Autodesk Fusion 360 part; units mm, degrees
(part 2 of 3)
  line L945 (31.8725, -23.9004) -> (31.8863, -23.9048)
  line L946 (31.8863, -23.9048) -> (31.9005, -23.9089)
  line L947 (31.9005, -23.9089) -> (31.9146, -23.9129)
  line L948 (31.9146, -23.9129) -> (31.9289, -23.9165)
  line L949 (31.9289, -23.9165) -> (31.9431, -23.9199)
  line L950 (31.9431, -23.9199) -> (31.9574, -23.9231)
  line L951 (31.9574, -23.9231) -> (31.9717, -23.9261)
  line L952 (31.9717, -23.9261) -> (31.986, -23.9287)
  line L953 (31.986, -23.9287) -> (32.0006, -23.9311)
  line L954 (32.0006, -23.9311) -> (32.0151, -23.9333)
  line L955 (32.0151, -23.9333) -> (32.0297, -23.9352)
  line L956 (32.0297, -23.9352) -> (32.0442, -23.9369)
  line L957 (32.0442, -23.9369) -> (32.0588, -23.9383)
  line L958 (32.0588, -23.9383) -> (32.0733, -23.9394)
  line L959 (32.0733, -23.9394) -> (32.0881, -23.9403)
  line L960 (32.0881, -23.9403) -> (32.1027, -23.941)
  line L961 (32.1027, -23.941) -> (32.1172, -23.9414)
  line L962 (32.1172, -23.9414) -> (32.1321, -23.9415)
  line L963 (32.1321, -23.9415) -> (57.3336, -23.9415)
  line L964 (57.3336, -23.9415) -> (57.3482, -23.9414)
  line L965 (-0.0202, 22.1566) -> (-0.0403, 22.1571)
  line L966 (-0.0403, 22.1571) -> (-0.0604, 22.158)
  line L967 (-0.0604, 22.158) -> (-0.0806, 22.1592)
  line L968 (-0.0806, 22.1592) -> (-0.1007, 22.1608)
  line L969 (-0.1007, 22.1608) -> (-0.1207, 22.1627)
  line L970 (-0.1207, 22.1627) -> (-0.1408, 22.165)
  line L971 (-0.1408, 22.165) -> (-0.1608, 22.1676)
  line L972 (-0.1608, 22.1676) -> (-0.1807, 22.1706)
  line L973 (-0.1807, 22.1706) -> (-0.2006, 22.1739)
  line L974 (-0.2006, 22.1739) -> (-0.2204, 22.1776)
  line L975 (-0.2204, 22.1776) -> (-0.2402, 22.1816)
  line L976 (-0.2402, 22.1816) -> (-0.2598, 22.186)
  line L977 (-0.2598, 22.186) -> (-0.2794, 22.1907)
  line L978 (-0.2794, 22.1907) -> (-0.299, 22.1957)
  line L979 (-0.299, 22.1957) -> (-0.3184, 22.2011)
  line L980 (-0.3184, 22.2011) -> (-0.3377, 22.2068)
  line L981 (-0.3377, 22.2068) -> (-0.3569, 22.2129)
  line L982 (-0.3569, 22.2129) -> (-0.3761, 22.2193)
  line L983 (-0.3761, 22.2193) -> (-0.3951, 22.226)
  line L984 (-0.3951, 22.226) -> (-0.4139, 22.2331)
  line L985 (-0.4139, 22.2331) -> (-0.4327, 22.2405)
  line L986 (-0.4327, 22.2405) -> (-0.4513, 22.2482)
  line L987 (-0.4513, 22.2482) -> (-0.4698, 22.2562)
  line L988 (-0.4698, 22.2562) -> (-0.4882, 22.2646)
  line L989 (-0.4882, 22.2646) -> (-0.5063, 22.2733)
  line L990 (-0.5063, 22.2733) -> (-0.5244, 22.2823)
  line L991 (-0.5244, 22.2823) -> (-0.5423, 22.2916)
  line L992 (-0.5423, 22.2916) -> (-0.56, 22.3012)
  line L993 (-0.56, 22.3012) -> (-0.5775, 22.3111)
  line L994 (-0.5775, 22.3111) -> (-0.5949, 22.3214)
  line L995 (-0.5949, 22.3214) -> (-0.6121, 22.3319)
  line L996 (-0.6121, 22.3319) -> (-0.6291, 22.3427)
  line L997 (-0.6291, 22.3427) -> (-0.6459, 22.3539)
  line L998 (-0.6459, 22.3539) -> (-0.6625, 22.3653)
  line L999 (-0.6625, 22.3653) -> (-0.6789, 22.377)
  line L1000 (-0.6789, 22.377) -> (-0.6951, 22.389)
  line L1001 (-0.6951, 22.389) -> (-0.7111, 22.4012)
  line L1002 (-0.7111, 22.4012) -> (-0.7269, 22.4138)
  line L1003 (-0.7269, 22.4138) -> (-0.7425, 22.4266)
  line L1004 (-0.7425, 22.4266) -> (-0.7578, 22.4397)
  line L1005 (-0.7578, 22.4397) -> (-0.7729, 22.4531)
  line L1006 (-0.7729, 22.4531) -> (-0.7878, 22.4667)
  line L1007 (-0.7878, 22.4667) -> (-0.8024, 22.4806)
  line L1008 (-0.8024, 22.4806) -> (-0.8168, 22.4947)
  line L1009 (-0.8168, 22.4947) -> (-0.8309, 22.5091)
  line L1010 (-0.8309, 22.5091) -> (-0.8448, 22.5237)
  line L1011 (-0.8448, 22.5237) -> (-0.8584, 22.5386)
  line L1012 (-0.8584, 22.5386) -> (-0.8717, 22.5536)
  line L1013 (-0.8717, 22.5536) -> (-0.8848, 22.569)
  line L1014 (-0.8848, 22.569) -> (-0.8977, 22.5845)
  line L1015 (-0.8977, 22.5845) -> (-0.9102, 22.6003)
  line L1016 (-0.9102, 22.6003) -> (-0.9225, 22.6163)
  line L1017 (-0.9225, 22.6163) -> (-0.9345, 22.6325)
  line L1018 (-0.9345, 22.6325) -> (-0.9462, 22.6489)
  line L1019 (-0.9462, 22.6489) -> (-0.9576, 22.6655)
  line L1020 (-0.9576, 22.6655) -> (-0.9687, 22.6823)
  line L1021 (-0.9687, 22.6823) -> (-0.9796, 22.6993)
  line L1022 (-0.9796, 22.6993) -> (-0.9901, 22.7165)
  line L1023 (-0.9901, 22.7165) -> (-1.0003, 22.7339)
  line L1024 (-1.0003, 22.7339) -> (-1.0102, 22.7514)
  line L1025 (-1.0102, 22.7514) -> (-1.0199, 22.7692)
  line L1026 (-1.0199, 22.7692) -> (-1.0292, 22.7871)
  line L1027 (-1.0292, 22.7871) -> (-1.0382, 22.8051)
  line L1028 (-1.0382, 22.8051) -> (-1.0468, 22.8233)
  line L1029 (-1.0468, 22.8233) -> (-1.0552, 22.8416)
  line L1030 (-1.0552, 22.8416) -> (-1.0632, 22.8601)
  line L1031 (-1.0632, 22.8601) -> (-1.071, 22.8788)
  line L1032 (-1.071, 22.8788) -> (-1.0783, 22.8975)
  line L1033 (-1.0783, 22.8975) -> (-1.0854, 22.9164)
  line L1034 (-1.0854, 22.9164) -> (-1.0921, 22.9354)
  line L1035 (-1.0921, 22.9354) -> (-1.0985, 22.9545)
  line L1036 (-1.0985, 22.9545) -> (-1.1046, 22.9737)
  line L1037 (-1.1046, 22.9737) -> (-1.1103, 22.9931)
  line L1038 (-1.1103, 22.9931) -> (-1.1157, 23.0125)
  line L1039 (-1.1157, 23.0125) -> (-1.1208, 23.032)
  line L1040 (-1.1208, 23.032) -> (-1.1255, 23.0516)
  line L1041 (-1.1255, 23.0516) -> (-1.1298, 23.0713)
  line L1042 (-1.1298, 23.0713) -> (-1.1339, 23.091)
  line L1043 (-1.1339, 23.091) -> (-1.1375, 23.1109)
  line L1044 (-1.1375, 23.1109) -> (-1.1408, 23.1307)
  line L1045 (-1.1408, 23.1307) -> (-1.1438, 23.1507)
  line L1046 (-1.1438, 23.1507) -> (-1.1465, 23.1707)
  line L1047 (-1.1465, 23.1707) -> (-1.1487, 23.1907)
  line L1048 (-1.1487, 23.1907) -> (-1.1507, 23.2108)
  line L1049 (-1.1507, 23.2108) -> (-1.1523, 23.2309)
  line L1050 (-1.1523, 23.2309) -> (-1.1535, 23.251)
  line L1051 (-1.1535, 23.251) -> (-1.1544, 23.2711)
  line L1052 (-1.1544, 23.2711) -> (-1.1549, 23.2913)
  line L1053 (-1.1549, 23.2913) -> (-1.1551, 23.3114)
  line L1054 (-1.1551, 23.3114) -> (-1.1549, 23.3316)
  line L1055 (-1.1549, 23.3316) -> (-1.1544, 23.3518)
  line L1056 (-1.1544, 23.3518) -> (-1.1535, 23.3719)
  line L1057 (-1.1535, 23.3719) -> (-1.1523, 23.392)
  line L1058 (-1.1523, 23.392) -> (-1.1507, 23.4121)
  line L1059 (-1.1507, 23.4121) -> (-1.1487, 23.4322)
  line L1060 (-1.1487, 23.4322) -> (-1.1465, 23.4522)
  line L1061 (-1.1465, 23.4522) -> (-1.1438, 23.4722)
  line L1062 (-1.1438, 23.4722) -> (-1.1408, 23.4921)
  line L1063 (-1.1408, 23.4921) -> (-1.1375, 23.512)
  line L1064 (-1.1375, 23.512) -> (-1.1339, 23.5318)
  line L1065 (-1.1339, 23.5318) -> (-1.1298, 23.5516)
  line L1066 (-1.1298, 23.5516) -> (-1.1255, 23.5713)
  line L1067 (-1.1255, 23.5713) -> (-1.1208, 23.5909)
  line L1068 (-1.1208, 23.5909) -> (-1.1157, 23.6104)
  line L1069 (-1.1157, 23.6104) -> (-1.1103, 23.6298)
  line L1070 (-1.1103, 23.6298) -> (-1.1046, 23.6491)
  line L1071 (-1.1046, 23.6491) -> (-1.0985, 23.6684)
  line L1072 (-1.0985, 23.6684) -> (-1.0921, 23.6875)
  line L1073 (-1.0921, 23.6875) -> (-1.0854, 23.7065)
  line L1074 (-1.0854, 23.7065) -> (-1.0783, 23.7254)
  line L1075 (-1.0783, 23.7254) -> (-1.071, 23.7441)
  line L1076 (-1.071, 23.7441) -> (-1.0632, 23.7628)
  line L1077 (-1.0632, 23.7628) -> (-1.0552, 23.7813)
  line L1078 (-1.0552, 23.7813) -> (-1.0468, 23.7996)
  line L1079 (-1.0468, 23.7996) -> (-1.0382, 23.8178)
  line L1080 (-1.0382, 23.8178) -> (-1.0292, 23.8358)
  line L1081 (-1.0292, 23.8358) -> (-1.0199, 23.8537)
  line L1082 (-1.0199, 23.8537) -> (-1.0102, 23.8714)
  line L1083 (-1.0102, 23.8714) -> (-1.0003, 23.889)
  line L1084 (-1.0003, 23.889) -> (-0.9901, 23.9063)
  line L1085 (-0.9901, 23.9063) -> (-0.9796, 23.9235)
  line L1086 (-0.9796, 23.9235) -> (-0.9687, 23.9405)
  line L1087 (-0.9687, 23.9405) -> (-0.9576, 23.9574)
  line L1088 (-0.9576, 23.9574) -> (-0.9462, 23.974)
  line L1089 (-0.9462, 23.974) -> (-0.9345, 23.9904)
  line L1090 (-0.9345, 23.9904) -> (-0.9225, 24.0066)
  line L1091 (-0.9225, 24.0066) -> (-0.9102, 24.0226)
  line L1092 (-0.9102, 24.0226) -> (-0.8977, 24.0383)
  line L1093 (-0.8977, 24.0383) -> (-0.8848, 24.0539)
  line L1094 (-0.8848, 24.0539) -> (-0.8717, 24.0693)
  line L1095 (-0.8717, 24.0693) -> (-0.8584, 24.0843)
  line L1096 (-0.8584, 24.0843) -> (-0.8448, 24.0992)
  line L1097 (-0.8448, 24.0992) -> (-0.8309, 24.1138)
  line L1098 (-0.8309, 24.1138) -> (-0.8168, 24.1282)
  line L1099 (-0.8168, 24.1282) -> (-0.8024, 24.1423)
  line L1100 (-0.8024, 24.1423) -> (-0.7878, 24.1562)
  line L1101 (-0.7878, 24.1562) -> (-0.7729, 24.1698)
  line L1102 (-0.7729, 24.1698) -> (-0.7578, 24.1832)
  line L1103 (-0.7578, 24.1832) -> (-0.7425, 24.1963)
  line L1104 (-0.7425, 24.1963) -> (-0.7269, 24.2091)
  line L1105 (-0.7269, 24.2091) -> (-0.7111, 24.2217)
  line L1106 (-0.7111, 24.2217) -> (-0.6951, 24.2339)
  line L1107 (-0.6951, 24.2339) -> (-0.6789, 24.2459)
  line L1108 (-0.6789, 24.2459) -> (-0.6625, 24.2576)
  line L1109 (-0.6625, 24.2576) -> (-0.6459, 24.269)
  line L1110 (-0.6459, 24.269) -> (-0.6291, 24.2802)
  line L1111 (-0.6291, 24.2802) -> (-0.6121, 24.291)
  line L1112 (-0.6121, 24.291) -> (-0.5949, 24.3015)
  line L1113 (-0.5949, 24.3015) -> (-0.5775, 24.3118)
  line L1114 (-0.5775, 24.3118) -> (-0.56, 24.3217)
  line L1115 (-0.56, 24.3217) -> (-0.5423, 24.3313)
  line L1116 (-0.5423, 24.3313) -> (-0.5244, 24.3406)
  line L1117 (-0.5244, 24.3406) -> (-0.5063, 24.3496)
  line L1118 (-0.5063, 24.3496) -> (-0.4882, 24.3583)
  line L1119 (-0.4882, 24.3583) -> (-0.4698, 24.3666)
  line L1120 (-0.4698, 24.3666) -> (-0.4513, 24.3747)
  line L1121 (-0.4513, 24.3747) -> (-0.4327, 24.3824)
  line L1122 (-0.4327, 24.3824) -> (-0.4139, 24.3898)
  line L1123 (-0.4139, 24.3898) -> (-0.3951, 24.3969)
  line L1124 (-0.3951, 24.3969) -> (-0.3761, 24.4036)
  line L1125 (-0.3761, 24.4036) -> (-0.3569, 24.41)
  line L1126 (-0.3569, 24.41) -> (-0.3377, 24.416)
  line L1127 (-0.3377, 24.416) -> (-0.3184, 24.4218)
  line L1128 (-0.3184, 24.4218) -> (-0.299, 24.4272)
  line L1129 (-0.299, 24.4272) -> (-0.2794, 24.4322)
  line L1130 (-0.2794, 24.4322) -> (-0.2598, 24.4369)
  line L1131 (-0.2598, 24.4369) -> (-0.2402, 24.4413)
  line L1132 (-0.2402, 24.4413) -> (-0.2204, 24.4453)
  line L1133 (-0.2204, 24.4453) -> (-0.2006, 24.449)
  line L1134 (-0.2006, 24.449) -> (-0.1807, 24.4523)
  line L1135 (-0.1807, 24.4523) -> (-0.1608, 24.4553)
  line L1136 (-0.1608, 24.4553) -> (-0.1408, 24.4579)
  line L1137 (-0.1408, 24.4579) -> (-0.1207, 24.4602)
  line L1138 (-0.1207, 24.4602) -> (-0.1007, 24.4621)
  line L1139 (-0.1007, 24.4621) -> (-0.0806, 24.4637)
  line L1140 (-0.0806, 24.4637) -> (-0.0604, 24.4649)
  line L1141 (-0.0604, 24.4649) -> (-0.0403, 24.4658)
  line L1142 (-0.0403, 24.4658) -> (-0.0202, 24.4663)
  line L1143 (-0.0202, 24.4663) -> (0, 24.4665)
  line L1144 (0, 24.4665) -> (0.0202, 24.4663)
  line L1145 (0.0202, 24.4663) -> (0.0403, 24.4658)
  line L1146 (0.0403, 24.4658) -> (0.0604, 24.4649)
  line L1147 (0.0604, 24.4649) -> (0.0806, 24.4637)
  line L1148 (0.0806, 24.4637) -> (0.1007, 24.4621)
  line L1149 (0.1007, 24.4621) -> (0.1207, 24.4602)
  line L1150 (0.1207, 24.4602) -> (0.1408, 24.4579)
  line L1151 (0.1408, 24.4579) -> (0.1608, 24.4553)
  line L1152 (0.1608, 24.4553) -> (0.1807, 24.4523)
  line L1153 (0.1807, 24.4523) -> (0.2006, 24.449)
  line L1154 (0.2006, 24.449) -> (0.2204, 24.4453)
  line L1155 (0.2204, 24.4453) -> (0.2402, 24.4413)
  line L1156 (0.2402, 24.4413) -> (0.2598, 24.4369)
  line L1157 (0.2598, 24.4369) -> (0.2794, 24.4322)
  line L1158 (0.2794, 24.4322) -> (0.299, 24.4272)
  line L1159 (0.299, 24.4272) -> (0.3184, 24.4218)
  line L1160 (0.3184, 24.4218) -> (0.3377, 24.416)
  line L1161 (0.3377, 24.416) -> (0.3569, 24.41)
  line L1162 (0.3569, 24.41) -> (0.3761, 24.4036)
  line L1163 (0.3761, 24.4036) -> (0.3951, 24.3969)
  line L1164 (0.3951, 24.3969) -> (0.4139, 24.3898)
  line L1165 (0.4139, 24.3898) -> (0.4327, 24.3824)
  line L1166 (0.4327, 24.3824) -> (0.4513, 24.3747)
  line L1167 (0.4513, 24.3747) -> (0.4698, 24.3666)
  line L1168 (0.4698, 24.3666) -> (0.4882, 24.3583)
  line L1169 (0.4882, 24.3583) -> (0.5063, 24.3496)
  line L1170 (0.5063, 24.3496) -> (0.5244, 24.3406)
  line L1171 (0.5244, 24.3406) -> (0.5423, 24.3313)
  line L1172 (0.5423, 24.3313) -> (0.56, 24.3217)
  line L1173 (0.56, 24.3217) -> (0.5775, 24.3118)
  line L1174 (0.5775, 24.3118) -> (0.5949, 24.3015)
  line L1175 (0.5949, 24.3015) -> (0.6121, 24.291)
  line L1176 (0.6121, 24.291) -> (0.6291, 24.2802)
  line L1177 (0.6291, 24.2802) -> (0.6459, 24.269)
  line L1178 (0.6459, 24.269) -> (0.6625, 24.2576)
  line L1179 (0.6625, 24.2576) -> (0.6789, 24.2459)
  line L1180 (0.6789, 24.2459) -> (0.6951, 24.2339)
  line L1181 (0.6951, 24.2339) -> (0.7111, 24.2217)
  line L1182 (0.7111, 24.2217) -> (0.7269, 24.2091)
  line L1183 (0.7269, 24.2091) -> (0.7425, 24.1963)
  line L1184 (0.7425, 24.1963) -> (0.7578, 24.1832)
  line L1185 (0.7578, 24.1832) -> (0.7729, 24.1698)
  line L1186 (0.7729, 24.1698) -> (0.7878, 24.1562)
  line L1187 (0.7878, 24.1562) -> (0.8024, 24.1423)
  line L1188 (0.8024, 24.1423) -> (0.8168, 24.1282)
  line L1189 (0.8168, 24.1282) -> (0.8309, 24.1138)
  line L1190 (0.8309, 24.1138) -> (0.8448, 24.0992)
  line L1191 (0.8448, 24.0992) -> (0.8584, 24.0843)
  line L1192 (0.8584, 24.0843) -> (0.8717, 24.0693)
  line L1193 (0.8717, 24.0693) -> (0.8848, 24.0539)
  line L1194 (0.8848, 24.0539) -> (0.8977, 24.0383)
  line L1195 (0.8977, 24.0383) -> (0.9102, 24.0226)
  line L1196 (0.9102, 24.0226) -> (0.9225, 24.0066)
  line L1197 (0.9225, 24.0066) -> (0.9345, 23.9904)
  line L1198 (0.9345, 23.9904) -> (0.9462, 23.974)
  line L1199 (0.9462, 23.974) -> (0.9576, 23.9574)
  line L1200 (0.9576, 23.9574) -> (0.9687, 23.9405)
  line L1201 (0.9687, 23.9405) -> (0.9796, 23.9235)
  line L1202 (0.9796, 23.9235) -> (0.9901, 23.9063)
  line L1203 (0.9901, 23.9063) -> (1.0003, 23.889)
  line L1204 (1.0003, 23.889) -> (1.0102, 23.8714)
  line L1205 (1.0102, 23.8714) -> (1.0199, 23.8537)
  line L1206 (1.0199, 23.8537) -> (1.0292, 23.8358)
  line L1207 (1.0292, 23.8358) -> (1.0382, 23.8178)
  line L1208 (1.0382, 23.8178) -> (1.0468, 23.7996)
  line L1209 (1.0468, 23.7996) -> (1.0552, 23.7813)
  line L1210 (1.0552, 23.7813) -> (1.0632, 23.7628)
  line L1211 (1.0632, 23.7628) -> (1.071, 23.7441)
  line L1212 (1.071, 23.7441) -> (1.0783, 23.7254)
  line L1213 (1.0783, 23.7254) -> (1.0854, 23.7065)
  line L1214 (1.0854, 23.7065) -> (1.0921, 23.6875)
  line L1215 (1.0921, 23.6875) -> (1.0985, 23.6684)
  line L1216 (1.0985, 23.6684) -> (1.1046, 23.6491)
  line L1217 (1.1046, 23.6491) -> (1.1103, 23.6298)
  line L1218 (1.1103, 23.6298) -> (1.1157, 23.6104)
  line L1219 (1.1157, 23.6104) -> (1.1208, 23.5909)
  line L1220 (1.1208, 23.5909) -> (1.1255, 23.5713)
  line L1221 (1.1255, 23.5713) -> (1.1298, 23.5516)
  line L1222 (1.1298, 23.5516) -> (1.1339, 23.5318)
  line L1223 (1.1339, 23.5318) -> (1.1375, 23.512)
  line L1224 (1.1375, 23.512) -> (1.1408, 23.4921)
  line L1225 (1.1408, 23.4921) -> (1.1438, 23.4722)
  line L1226 (1.1438, 23.4722) -> (1.1465, 23.4522)
  line L1227 (1.1465, 23.4522) -> (1.1487, 23.4322)
  line L1228 (1.1487, 23.4322) -> (1.1507, 23.4121)
  line L1229 (1.1507, 23.4121) -> (1.1523, 23.392)
  line L1230 (1.1523, 23.392) -> (1.1535, 23.3719)
  line L1231 (1.1535, 23.3719) -> (1.1544, 23.3518)
  line L1232 (1.1544, 23.3518) -> (1.1549, 23.3316)
  line L1233 (1.1549, 23.3316) -> (1.1551, 23.3114)
  line L1234 (1.1551, 23.3114) -> (1.1549, 23.2913)
  line L1235 (1.1549, 23.2913) -> (1.1544, 23.2711)
  line L1236 (1.1544, 23.2711) -> (1.1535, 23.251)
  line L1237 (1.1535, 23.251) -> (1.1523, 23.2309)
  line L1238 (1.1523, 23.2309) -> (1.1507, 23.2108)
  line L1239 (1.1507, 23.2108) -> (1.1487, 23.1907)
  line L1240 (1.1487, 23.1907) -> (1.1465, 23.1707)
  line L1241 (1.1465, 23.1707) -> (1.1438, 23.1507)
  line L1242 (1.1438, 23.1507) -> (1.1408, 23.1307)
  line L1243 (1.1408, 23.1307) -> (1.1375, 23.1109)
  line L1244 (1.1375, 23.1109) -> (1.1339, 23.091)
  line L1245 (1.1339, 23.091) -> (1.1298, 23.0713)
  line L1246 (1.1298, 23.0713) -> (1.1255, 23.0516)
  line L1247 (1.1255, 23.0516) -> (1.1208, 23.032)
  line L1248 (1.1208, 23.032) -> (1.1157, 23.0125)
  line L1249 (1.1157, 23.0125) -> (1.1103, 22.9931)
  line L1250 (1.1103, 22.9931) -> (1.1046, 22.9737)
  line L1251 (1.1046, 22.9737) -> (1.0985, 22.9545)
  line L1252 (1.0985, 22.9545) -> (1.0921, 22.9354)
  line L1253 (1.0921, 22.9354) -> (1.0854, 22.9164)
  line L1254 (1.0854, 22.9164) -> (1.0783, 22.8975)
  line L1255 (1.0783, 22.8975) -> (1.071, 22.8788)
  line L1256 (1.071, 22.8788) -> (1.0632, 22.8601)
  line L1257 (1.0632, 22.8601) -> (1.0552, 22.8416)
  line L1258 (1.0552, 22.8416) -> (1.0468, 22.8233)
  line L1259 (1.0468, 22.8233) -> (1.0382, 22.8051)
  line L1260 (1.0382, 22.8051) -> (1.0292, 22.7871)
  line L1261 (1.0292, 22.7871) -> (1.0199, 22.7692)
  line L1262 (1.0199, 22.7692) -> (1.0102, 22.7514)
  line L1263 (1.0102, 22.7514) -> (1.0003, 22.7339)
  line L1264 (1.0003, 22.7339) -> (0.9901, 22.7165)
  line L1265 (0.9901, 22.7165) -> (0.9796, 22.6993)
  line L1266 (0.9796, 22.6993) -> (0.9687, 22.6823)
  line L1267 (0.9687, 22.6823) -> (0.9576, 22.6655)
  line L1268 (0.9576, 22.6655) -> (0.9462, 22.6489)
  line L1269 (0.9462, 22.6489) -> (0.9345, 22.6325)
  line L1270 (0.9345, 22.6325) -> (0.9225, 22.6163)
  line L1271 (0.9225, 22.6163) -> (0.9102, 22.6003)
  line L1272 (0.9102, 22.6003) -> (0.8977, 22.5845)
  line L1273 (0.8977, 22.5845) -> (0.8848, 22.569)
  line L1274 (0.8848, 22.569) -> (0.8717, 22.5536)
  line L1275 (0.8717, 22.5536) -> (0.8584, 22.5386)
  line L1276 (0.8584, 22.5386) -> (0.8448, 22.5237)
  line L1277 (0.8448, 22.5237) -> (0.8309, 22.5091)
  line L1278 (0.8309, 22.5091) -> (0.8168, 22.4947)
  line L1279 (0.8168, 22.4947) -> (0.8024, 22.4806)
  line L1280 (0.8024, 22.4806) -> (0.7878, 22.4667)
  line L1281 (0.7878, 22.4667) -> (0.7729, 22.4531)
  line L1282 (0.7729, 22.4531) -> (0.7578, 22.4397)
  line L1283 (0.7578, 22.4397) -> (0.7425, 22.4266)
  line L1284 (0.7425, 22.4266) -> (0.7269, 22.4138)
  line L1285 (0.7269, 22.4138) -> (0.7111, 22.4012)
  line L1286 (0.7111, 22.4012) -> (0.6951, 22.389)
  line L1287 (0.6951, 22.389) -> (0.6789, 22.377)
  line L1288 (0.6789, 22.377) -> (0.6625, 22.3653)
  line L1289 (0.6625, 22.3653) -> (0.6459, 22.3539)
  line L1290 (0.6459, 22.3539) -> (0.6291, 22.3427)
  line L1291 (0.6291, 22.3427) -> (0.6121, 22.3319)
  line L1292 (0.6121, 22.3319) -> (0.5949, 22.3214)
  line L1293 (0.5949, 22.3214) -> (0.5775, 22.3111)
  line L1294 (0.5775, 22.3111) -> (0.56, 22.3012)
  line L1295 (0.56, 22.3012) -> (0.5423, 22.2916)
  line L1296 (0.5423, 22.2916) -> (0.5244, 22.2823)
  line L1297 (0.5244, 22.2823) -> (0.5063, 22.2733)
  line L1298 (0.5063, 22.2733) -> (0.4882, 22.2646)
  line L1299 (0.4882, 22.2646) -> (0.4698, 22.2562)
  line L1300 (0.4698, 22.2562) -> (0.4513, 22.2482)
  line L1301 (0.4513, 22.2482) -> (0.4327, 22.2405)
  line L1302 (0.4327, 22.2405) -> (0.4139, 22.2331)
  line L1303 (0.4139, 22.2331) -> (0.3951, 22.226)
  line L1304 (0.3951, 22.226) -> (0.3761, 22.2193)
  line L1305 (0.3761, 22.2193) -> (0.3569, 22.2129)
  line L1306 (0.3569, 22.2129) -> (0.3377, 22.2068)
  line L1307 (0.3377, 22.2068) -> (0.3184, 22.2011)
  line L1308 (0.3184, 22.2011) -> (0.299, 22.1957)
  line L1309 (0.299, 22.1957) -> (0.2794, 22.1907)
  line L1310 (0.2794, 22.1907) -> (0.2598, 22.186)
  line L1311 (0.2598, 22.186) -> (0.2402, 22.1816)
  line L1312 (0.2402, 22.1816) -> (0.2204, 22.1776)
  line L1313 (0.2204, 22.1776) -> (0.2006, 22.1739)
  line L1314 (0.2006, 22.1739) -> (0.1807, 22.1706)
  line L1315 (0.1807, 22.1706) -> (0.1608, 22.1676)
  line L1316 (0.1608, 22.1676) -> (0.1408, 22.165)
  line L1317 (0.1408, 22.165) -> (0.1207, 22.1627)
  line L1318 (0.1207, 22.1627) -> (0.1007, 22.1608)
  line L1319 (0.1007, 22.1608) -> (0.0806, 22.1592)
  line L1320 (0.0806, 22.1592) -> (0.0604, 22.158)
  line L1321 (0.0604, 22.158) -> (0.0403, 22.1571)
  line L1322 (0.0403, 22.1571) -> (0.0202, 22.1566)
  line L1323 (0.0202, 22.1566) -> (0, 22.1564)
  line L1324 (0, 22.1564) -> (-0.0202, 22.1566)
  line L1325 (34.6321, 22.1566) -> (34.6117, 22.1571)
  line L1326 (34.6117, 22.1571) -> (34.5916, 22.158)
  line L1327 (34.5916, 22.158) -> (34.5715, 22.1592)
  line L1328 (34.5715, 22.1592) -> (34.5514, 22.1608)
  line L1329 (34.5514, 22.1608) -> (34.5313, 22.1627)
  line L1330 (34.5313, 22.1627) -> (34.5115, 22.165)
  line L1331 (34.5115, 22.165) -> (34.4913, 22.1676)
  line L1332 (34.4913, 22.1676) -> (34.4715, 22.1706)
  line L1333 (34.4715, 22.1706) -> (34.4517, 22.1739)
  line L1334 (34.4517, 22.1739) -> (34.4318, 22.1776)
  line L1335 (34.4318, 22.1776) -> (34.412, 22.1816)
  line L1336 (34.412, 22.1816) -> (34.3924, 22.186)
  line L1337 (34.3924, 22.186) -> (34.3728, 22.1907)
  line L1338 (34.3728, 22.1907) -> (34.3532, 22.1957)
  line L1339 (34.3532, 22.1957) -> (34.3337, 22.2011)
  line L1340 (34.3337, 22.2011) -> (34.3143, 22.2068)
  line L1341 (34.3143, 22.2068) -> (34.2953, 22.2129)
  line L1342 (34.2953, 22.2129) -> (34.276, 22.2193)
  line L1343 (34.276, 22.2193) -> (34.2572, 22.226)
  line L1344 (34.2572, 22.226) -> (34.2381, 22.2331)
  line L1345 (34.2381, 22.2331) -> (34.2194, 22.2405)
  line L1346 (34.2194, 22.2405) -> (34.2008, 22.2482)
  line L1347 (34.2008, 22.2482) -> (34.1823, 22.2562)
  line L1348 (34.1823, 22.2562) -> (34.1641, 22.2646)
  line L1349 (34.1641, 22.2646) -> (34.1458, 22.2733)
  line L1350 (34.1458, 22.2733) -> (34.1278, 22.2823)
  line L1351 (34.1278, 22.2823) -> (34.1098, 22.2916)
  line L1352 (34.1098, 22.2916) -> (34.0921, 22.3012)
  line L1353 (34.0921, 22.3012) -> (34.0746, 22.3111)
  line L1354 (34.0746, 22.3111) -> (34.0572, 22.3214)
  line L1355 (34.0572, 22.3214) -> (34.04, 22.3319)
  line L1356 (34.04, 22.3319) -> (34.023, 22.3427)
  line L1357 (34.023, 22.3427) -> (34.0064, 22.3539)
  line L1358 (34.0064, 22.3539) -> (33.9897, 22.3653)
  line L1359 (33.9897, 22.3653) -> (33.9733, 22.377)
  line L1360 (33.9733, 22.377) -> (33.9569, 22.389)
  line L1361 (33.9569, 22.389) -> (33.941, 22.4012)
  line L1362 (33.941, 22.4012) -> (33.9251, 22.4138)
  line L1363 (33.9251, 22.4138) -> (33.9098, 22.4266)
  line L1364 (33.9098, 22.4266) -> (33.8944, 22.4397)
  line L1365 (33.8944, 22.4397) -> (33.8794, 22.4531)
  line L1366 (33.8794, 22.4531) -> (33.8643, 22.4667)
  line L1367 (33.8643, 22.4667) -> (33.8497, 22.4806)
  line L1368 (33.8497, 22.4806) -> (33.8354, 22.4947)
  line L1369 (33.8354, 22.4947) -> (33.8212, 22.5091)
  line L1370 (33.8212, 22.5091) -> (33.8074, 22.5237)
  line L1371 (33.8074, 22.5237) -> (33.7936, 22.5386)
  line L1372 (33.7936, 22.5386) -> (33.7804, 22.5536)
  line L1373 (33.7804, 22.5536) -> (33.7672, 22.569)
  line L1374 (33.7672, 22.569) -> (33.7545, 22.5845)
  line L1375 (33.7545, 22.5845) -> (33.742, 22.6003)
  line L1376 (33.742, 22.6003) -> (33.7296, 22.6163)
  line L1377 (33.7296, 22.6163) -> (33.7177, 22.6325)
  line L1378 (33.7177, 22.6325) -> (33.7061, 22.6489)
  line L1379 (33.7061, 22.6489) -> (33.6944, 22.6655)
  line L1380 (33.6944, 22.6655) -> (33.6833, 22.6823)
  line L1381 (33.6833, 22.6823) -> (33.6725, 22.6993)
  line L1382 (33.6725, 22.6993) -> (33.6621, 22.7165)
  line L1383 (33.6621, 22.7165) -> (33.6518, 22.7339)
  line L1384 (33.6518, 22.7339) -> (33.6418, 22.7514)
  line L1385 (33.6418, 22.7514) -> (33.6322, 22.7692)
  line L1386 (33.6322, 22.7692) -> (33.623, 22.7871)
  line L1387 (33.623, 22.7871) -> (33.614, 22.8051)
  line L1388 (33.614, 22.8051) -> (33.6053, 22.8233)
  line L1389 (33.6053, 22.8233) -> (33.5971, 22.8416)
  line L1390 (33.5971, 22.8416) -> (33.5889, 22.8601)
  line L1391 (33.5889, 22.8601) -> (33.5812, 22.8788)
  line L1392 (33.5812, 22.8788) -> (33.5738, 22.8975)
  line L1393 (33.5738, 22.8975) -> (33.5666, 22.9164)
  line L1394 (33.5666, 22.9164) -> (33.56, 22.9354)
  line L1395 (33.56, 22.9354) -> (33.5537, 22.9545)
  line L1396 (33.5537, 22.9545) -> (33.5476, 22.9737)
  line L1397 (33.5476, 22.9737) -> (33.5418, 22.9931)
  line L1398 (33.5418, 22.9931) -> (33.5365, 23.0125)
  line L1399 (33.5365, 23.0125) -> (33.5314, 23.032)
  line L1400 (33.5314, 23.032) -> (33.5267, 23.0516)
  line L1401 (33.5267, 23.0516) -> (33.5224, 23.0713)
  line L1402 (33.5224, 23.0713) -> (33.5182, 23.091)
  line L1403 (33.5182, 23.091) -> (33.5145, 23.1109)
  line L1404 (33.5145, 23.1109) -> (33.5113, 23.1307)
  line L1405 (33.5113, 23.1307) -> (33.5084, 23.1507)
  line L1406 (33.5084, 23.1507) -> (33.5058, 23.1707)
  line L1407 (33.5058, 23.1707) -> (33.5034, 23.1907)
  line L1408 (33.5034, 23.1907) -> (33.5015, 23.2108)
  line L1409 (33.5015, 23.2108) -> (33.5, 23.2309)
  line L1410 (33.5, 23.2309) -> (33.4986, 23.251)
  line L1411 (33.4986, 23.251) -> (33.4978, 23.2711)
  line L1412 (33.4978, 23.2711) -> (33.4973, 23.2913)
  line L1413 (33.4973, 23.2913) -> (33.497, 23.3114)
  line L1414 (33.497, 23.3114) -> (33.4973, 23.3316)
  line L1415 (33.4973, 23.3316) -> (33.4978, 23.3518)
  line L1416 (33.4978, 23.3518) -> (33.4986, 23.3719)
  line L1417 (33.4986, 23.3719) -> (33.5, 23.392)
  line L1418 (33.5, 23.392) -> (33.5015, 23.4121)
  line L1419 (33.5015, 23.4121) -> (33.5034, 23.4322)
  line L1420 (33.5034, 23.4322) -> (33.5058, 23.4522)
  line L1421 (33.5058, 23.4522) -> (33.5084, 23.4722)
  line L1422 (33.5084, 23.4722) -> (33.5113, 23.4921)
  line L1423 (33.5113, 23.4921) -> (33.5145, 23.512)
  line L1424 (33.5145, 23.512) -> (33.5182, 23.5318)
  line L1425 (33.5182, 23.5318) -> (33.5224, 23.5516)
  line L1426 (33.5224, 23.5516) -> (33.5267, 23.5713)
  line L1427 (33.5267, 23.5713) -> (33.5314, 23.5909)
  line L1428 (33.5314, 23.5909) -> (33.5365, 23.6104)
  line L1429 (33.5365, 23.6104) -> (33.5418, 23.6298)
  line L1430 (33.5418, 23.6298) -> (33.5476, 23.6491)
  line L1431 (33.5476, 23.6491) -> (33.5537, 23.6684)
  line L1432 (33.5537, 23.6684) -> (33.56, 23.6875)
  line L1433 (33.56, 23.6875) -> (33.5666, 23.7065)
  line L1434 (33.5666, 23.7065) -> (33.5738, 23.7254)
  line L1435 (33.5738, 23.7254) -> (33.5812, 23.7441)
  line L1436 (33.5812, 23.7441) -> (33.5889, 23.7628)
  line L1437 (33.5889, 23.7628) -> (33.5971, 23.7813)
  line L1438 (33.5971, 23.7813) -> (33.6053, 23.7996)
  line L1439 (33.6053, 23.7996) -> (33.614, 23.8178)
  line L1440 (33.614, 23.8178) -> (33.623, 23.8358)
  line L1441 (33.623, 23.8358) -> (33.6322, 23.8537)
  line L1442 (33.6322, 23.8537) -> (33.6418, 23.8714)
  line L1443 (33.6418, 23.8714) -> (33.6518, 23.889)
  line L1444 (33.6518, 23.889) -> (33.6621, 23.9063)
  line L1445 (33.6621, 23.9063) -> (33.6725, 23.9235)
  line L1446 (33.6725, 23.9235) -> (33.6833, 23.9405)
  line L1447 (33.6833, 23.9405) -> (33.6944, 23.9574)
  line L1448 (33.6944, 23.9574) -> (33.7061, 23.974)
  line L1449 (33.7061, 23.974) -> (33.7177, 23.9904)
  line L1450 (33.7177, 23.9904) -> (33.7296, 24.0066)
  line L1451 (33.7296, 24.0066) -> (33.742, 24.0226)
  line L1452 (33.742, 24.0226) -> (33.7545, 24.0383)
  line L1453 (33.7545, 24.0383) -> (33.7672, 24.0539)
  line L1454 (33.7672, 24.0539) -> (33.7804, 24.0693)
  line L1455 (33.7804, 24.0693) -> (33.7936, 24.0843)
  line L1456 (33.7936, 24.0843) -> (33.8074, 24.0992)
  line L1457 (33.8074, 24.0992) -> (33.8212, 24.1138)
  line L1458 (33.8212, 24.1138) -> (33.8354, 24.1282)
  line L1459 (33.8354, 24.1282) -> (33.8497, 24.1423)
  line L1460 (33.8497, 24.1423) -> (33.8643, 24.1562)
  line L1461 (33.8643, 24.1562) -> (33.8794, 24.1698)
  line L1462 (33.8794, 24.1698) -> (33.8944, 24.1832)
  line L1463 (33.8944, 24.1832) -> (33.9098, 24.1963)
  line L1464 (33.9098, 24.1963) -> (33.9251, 24.2091)
  line L1465 (33.9251, 24.2091) -> (33.941, 24.2217)
  line L1466 (33.941, 24.2217) -> (33.9569, 24.2339)
  line L1467 (33.9569, 24.2339) -> (33.9733, 24.2459)
  line L1468 (33.9733, 24.2459) -> (33.9897, 24.2576)
  line L1469 (33.9897, 24.2576) -> (34.0064, 24.269)
  line L1470 (34.0064, 24.269) -> (34.023, 24.2802)
  line L1471 (34.023, 24.2802) -> (34.04, 24.291)
  line L1472 (34.04, 24.291) -> (34.0572, 24.3015)
  line L1473 (34.0572, 24.3015) -> (34.0746, 24.3118)
  line L1474 (34.0746, 24.3118) -> (34.0921, 24.3217)
  line L1475 (34.0921, 24.3217) -> (34.1098, 24.3313)
  line L1476 (34.1098, 24.3313) -> (34.1278, 24.3406)
  line L1477 (34.1278, 24.3406) -> (34.1458, 24.3496)
  line L1478 (34.1458, 24.3496) -> (34.1641, 24.3583)
  line L1479 (34.1641, 24.3583) -> (34.1823, 24.3666)
  line L1480 (34.1823, 24.3666) -> (34.2008, 24.3747)
  line L1481 (34.2008, 24.3747) -> (34.2194, 24.3824)
  line L1482 (34.2194, 24.3824) -> (34.2381, 24.3898)
  line L1483 (34.2381, 24.3898) -> (34.2572, 24.3969)
  line L1484 (34.2572, 24.3969) -> (34.276, 24.4036)
  line L1485 (34.276, 24.4036) -> (34.2953, 24.41)
  line L1486 (34.2953, 24.41) -> (34.3143, 24.416)
  line L1487 (34.3143, 24.416) -> (34.3337, 24.4218)
  line L1488 (34.3337, 24.4218) -> (34.3532, 24.4272)
  line L1489 (34.3532, 24.4272) -> (34.3728, 24.4322)
  line L1490 (34.3728, 24.4322) -> (34.3924, 24.4369)
  line L1491 (34.3924, 24.4369) -> (34.412, 24.4413)
  line L1492 (34.412, 24.4413) -> (34.4318, 24.4453)
  line L1493 (34.4318, 24.4453) -> (34.4517, 24.449)
  line L1494 (34.4517, 24.449) -> (34.4715, 24.4523)
  line L1495 (34.4715, 24.4523) -> (34.4913, 24.4553)
  line L1496 (34.4913, 24.4553) -> (34.5115, 24.4579)
  line L1497 (34.5115, 24.4579) -> (34.5313, 24.4602)
  line L1498 (34.5313, 24.4602) -> (34.5514, 24.4621)
  line L1499 (34.5514, 24.4621) -> (34.5715, 24.4637)
  line L1500 (34.5715, 24.4637) -> (34.5916, 24.4649)
  line L1501 (34.5916, 24.4649) -> (34.6117, 24.4658)
  line L1502 (34.6117, 24.4658) -> (34.6321, 24.4663)
  line L1503 (34.6321, 24.4663) -> (34.6522, 24.4665)
  line L1504 (34.6522, 24.4665) -> (34.6723, 24.4663)
  line L1505 (34.6723, 24.4663) -> (34.6924, 24.4658)
  line L1506 (34.6924, 24.4658) -> (34.7125, 24.4649)
  line L1507 (34.7125, 24.4649) -> (34.7326, 24.4637)
  line L1508 (34.7326, 24.4637) -> (34.7528, 24.4621)
  line L1509 (34.7528, 24.4621) -> (34.7729, 24.4602)
  line L1510 (34.7729, 24.4602) -> (34.793, 24.4579)
  line L1511 (34.793, 24.4579) -> (34.8128, 24.4553)
  line L1512 (34.8128, 24.4553) -> (34.8329, 24.4523)
  line L1513 (34.8329, 24.4523) -> (34.8528, 24.449)
  line L1514 (34.8528, 24.449) -> (34.8726, 24.4453)
  line L1515 (34.8726, 24.4453) -> (34.8922, 24.4413)
  line L1516 (34.8922, 24.4413) -> (34.912, 24.4369)
  line L1517 (34.912, 24.4369) -> (34.9316, 24.4322)
  line L1518 (34.9316, 24.4322) -> (34.9512, 24.4272)
  line L1519 (34.9512, 24.4272) -> (34.9705, 24.4218)
  line L1520 (34.9705, 24.4218) -> (34.9898, 24.416)
  line L1521 (34.9898, 24.416) -> (35.0091, 24.41)
  line L1522 (35.0091, 24.41) -> (35.0282, 24.4036)
  line L1523 (35.0282, 24.4036) -> (35.0472, 24.3969)
  line L1524 (35.0472, 24.3969) -> (35.066, 24.3898)
  line L1525 (35.066, 24.3898) -> (35.0848, 24.3824)
  line L1526 (35.0848, 24.3824) -> (35.1036, 24.3747)
  line L1527 (35.1036, 24.3747) -> (35.1219, 24.3666)
  line L1528 (35.1219, 24.3666) -> (35.1404, 24.3583)
  line L1529 (35.1404, 24.3583) -> (35.1586, 24.3496)
  line L1530 (35.1586, 24.3496) -> (35.1766, 24.3406)
  line L1531 (35.1766, 24.3406) -> (35.1943, 24.3313)
  line L1532 (35.1943, 24.3313) -> (35.2121, 24.3217)
  line L1533 (35.2121, 24.3217) -> (35.2298, 24.3118)
  line L1534 (35.2298, 24.3118) -> (35.247, 24.3015)
  line L1535 (35.247, 24.3015) -> (35.2642, 24.291)
  line L1536 (35.2642, 24.291) -> (35.2811, 24.2802)
  line L1537 (35.2811, 24.2802) -> (35.2981, 24.269)
  line L1538 (35.2981, 24.269) -> (35.3147, 24.2576)
  line L1539 (35.3147, 24.2576) -> (35.3311, 24.2459)
  line L1540 (35.3311, 24.2459) -> (35.3473, 24.2339)
  line L1541 (35.3473, 24.2339) -> (35.3632, 24.2217)
  line L1542 (35.3632, 24.2217) -> (35.379, 24.2091)
  line L1543 (35.379, 24.2091) -> (35.3946, 24.1963)
  line L1544 (35.3946, 24.1963) -> (35.41, 24.1832)
  line L1545 (35.41, 24.1832) -> (35.4251, 24.1698)
  line L1546 (35.4251, 24.1698) -> (35.4399, 24.1562)
  line L1547 (35.4399, 24.1562) -> (35.4544, 24.1423)
  line L1548 (35.4544, 24.1423) -> (35.469, 24.1282)
  line L1549 (35.469, 24.1282) -> (35.483, 24.1138)
  line L1550 (35.483, 24.1138) -> (35.497, 24.0992)
  line L1551 (35.497, 24.0992) -> (35.5105, 24.0843)
  line L1552 (35.5105, 24.0843) -> (35.524, 24.0693)
  line L1553 (35.524, 24.0693) -> (35.537, 24.0539)
  line L1554 (35.537, 24.0539) -> (35.5497, 24.0383)
  line L1555 (35.5497, 24.0383) -> (35.5624, 24.0226)
  line L1556 (35.5624, 24.0226) -> (35.5746, 24.0066)
  line L1557 (35.5746, 24.0066) -> (35.5867, 23.9904)
  line L1558 (35.5867, 23.9904) -> (35.5984, 23.974)
  line L1559 (35.5984, 23.974) -> (35.6097, 23.9574)
  line L1560 (35.6097, 23.9574) -> (35.6209, 23.9405)
  line L1561 (35.6209, 23.9405) -> (35.6317, 23.9235)
  line L1562 (35.6317, 23.9235) -> (35.6423, 23.9063)
  line L1563 (35.6423, 23.9063) -> (35.6523, 23.889)
  line L1564 (35.6523, 23.889) -> (35.6624, 23.8714)
  line L1565 (35.6624, 23.8714) -> (35.6719, 23.8537)
  line L1566 (35.6719, 23.8537) -> (35.6814, 23.8358)
  line L1567 (35.6814, 23.8358) -> (35.6904, 23.8178)
  line L1568 (35.6904, 23.8178) -> (35.6989, 23.7996)
  line L1569 (35.6989, 23.7996) -> (35.7074, 23.7813)
  line L1570 (35.7074, 23.7813) -> (35.7153, 23.7628)
  line L1571 (35.7153, 23.7628) -> (35.723, 23.7441)
  line L1572 (35.723, 23.7441) -> (35.7304, 23.7254)
  line L1573 (35.7304, 23.7254) -> (35.7375, 23.7065)
  line L1574 (35.7375, 23.7065) -> (35.7444, 23.6875)
  line L1575 (35.7444, 23.6875) -> (35.7508, 23.6684)
  line L1576 (35.7508, 23.6684) -> (35.7568, 23.6491)
  line L1577 (35.7568, 23.6491) -> (35.7624, 23.6298)
  line L1578 (35.7624, 23.6298) -> (35.768, 23.6104)
  line L1579 (35.768, 23.6104) -> (35.773, 23.5909)
  line L1580 (35.773, 23.5909) -> (35.7775, 23.5713)
  line L1581 (35.7775, 23.5713) -> (35.782, 23.5516)
  line L1582 (35.782, 23.5516) -> (35.786, 23.5318)
  line L1583 (35.786, 23.5318) -> (35.7897, 23.512)
  line L1584 (35.7897, 23.512) -> (35.7931, 23.4921)
  line L1585 (35.7931, 23.4921) -> (35.796, 23.4722)
  line L1586 (35.796, 23.4722) -> (35.7987, 23.4522)
  line L1587 (35.7987, 23.4522) -> (35.8008, 23.4322)
  line L1588 (35.8008, 23.4322) -> (35.8029, 23.4121)
  line L1589 (35.8029, 23.4121) -> (35.8045, 23.392)
  line L1590 (35.8045, 23.392) -> (35.8055, 23.3719)
  line L1591 (35.8055, 23.3719) -> (35.8066, 23.3518)
  line L1592 (35.8066, 23.3518) -> (35.8071, 23.3316)
  line L1593 (35.8071, 23.3316) -> (35.8071, 23.3114)
  line L1594 (35.8071, 23.3114) -> (35.8071, 23.2913)
  line L1595 (35.8071, 23.2913) -> (35.8066, 23.2711)
  line L1596 (35.8066, 23.2711) -> (35.8055, 23.251)
  line L1597 (35.8055, 23.251) -> (35.8045, 23.2309)
  line L1598 (35.8045, 23.2309) -> (35.8029, 23.2108)
  line L1599 (35.8029, 23.2108) -> (35.8008, 23.1907)
  line L1600 (35.8008, 23.1907) -> (35.7987, 23.1707)
  line L1601 (35.7987, 23.1707) -> (35.796, 23.1507)
  line L1602 (35.796, 23.1507) -> (35.7931, 23.1307)
  line L1603 (35.7931, 23.1307) -> (35.7897, 23.1109)
  line L1604 (35.7897, 23.1109) -> (35.786, 23.091)
  line L1605 (35.786, 23.091) -> (35.782, 23.0713)
  line L1606 (35.782, 23.0713) -> (35.7775, 23.0516)
  line L1607 (35.7775, 23.0516) -> (35.773, 23.032)
  line L1608 (35.773, 23.032) -> (35.768, 23.0125)
  line L1609 (35.768, 23.0125) -> (35.7624, 22.9931)
  line L1610 (35.7624, 22.9931) -> (35.7568, 22.9737)
  line L1611 (35.7568, 22.9737) -> (35.7508, 22.9545)
  line L1612 (35.7508, 22.9545) -> (35.7444, 22.9354)
  line L1613 (35.7444, 22.9354) -> (35.7375, 22.9164)
  line L1614 (35.7375, 22.9164) -> (35.7304, 22.8975)
  line L1615 (35.7304, 22.8975) -> (35.723, 22.8788)
  line L1616 (35.723, 22.8788) -> (35.7153, 22.8601)
  line L1617 (35.7153, 22.8601) -> (35.7074, 22.8416)
  line L1618 (35.7074, 22.8416) -> (35.6989, 22.8233)
  line L1619 (35.6989, 22.8233) -> (35.6904, 22.8051)
  line L1620 (35.6904, 22.8051) -> (35.6814, 22.7871)
  line L1621 (35.6814, 22.7871) -> (35.6719, 22.7692)
  line L1622 (35.6719, 22.7692) -> (35.6624, 22.7514)
  line L1623 (35.6624, 22.7514) -> (35.6523, 22.7339)
  line L1624 (35.6523, 22.7339) -> (35.6423, 22.7165)
  line L1625 (35.6423, 22.7165) -> (35.6317, 22.6993)
  line L1626 (35.6317, 22.6993) -> (35.6209, 22.6823)
  line L1627 (35.6209, 22.6823) -> (35.6097, 22.6655)
  line L1628 (35.6097, 22.6655) -> (35.5984, 22.6489)
  line L1629 (35.5984, 22.6489) -> (35.5867, 22.6325)
  line L1630 (35.5867, 22.6325) -> (35.5746, 22.6163)
  line L1631 (35.5746, 22.6163) -> (35.5624, 22.6003)
  line L1632 (35.5624, 22.6003) -> (35.5497, 22.5845)
  line L1633 (35.5497, 22.5845) -> (35.537, 22.569)
  line L1634 (35.537, 22.569) -> (35.524, 22.5536)
  line L1635 (35.524, 22.5536) -> (35.5105, 22.5386)
  line L1636 (35.5105, 22.5386) -> (35.497, 22.5237)
  line L1637 (35.497, 22.5237) -> (35.483, 22.5091)
  line L1638 (35.483, 22.5091) -> (35.469, 22.4947)
  line L1639 (35.469, 22.4947) -> (35.4544, 22.4806)
  line L1640 (35.4544, 22.4806) -> (35.4399, 22.4667)
  line L1641 (35.4399, 22.4667) -> (35.4251, 22.4531)
  line L1642 (35.4251, 22.4531) -> (35.41, 22.4397)
  line L1643 (35.41, 22.4397) -> (35.3946, 22.4266)
  line L1644 (35.3946, 22.4266) -> (35.379, 22.4138)
  line L1645 (35.379, 22.4138) -> (35.3632, 22.4012)
  line L1646 (35.3632, 22.4012) -> (35.3473, 22.389)
  line L1647 (35.3473, 22.389) -> (35.3311, 22.377)
  line L1648 (35.3311, 22.377) -> (35.3147, 22.3653)
  line L1649 (35.3147, 22.3653) -> (35.2981, 22.3539)
  line L1650 (35.2981, 22.3539) -> (35.2811, 22.3427)
  line L1651 (35.2811, 22.3427) -> (35.2642, 22.3319)
  line L1652 (35.2642, 22.3319) -> (35.247, 22.3214)
  line L1653 (35.247, 22.3214) -> (35.2298, 22.3111)
  line L1654 (35.2298, 22.3111) -> (35.2121, 22.3012)
  line L1655 (35.2121, 22.3012) -> (35.1943, 22.2916)
  line L1656 (35.1943, 22.2916) -> (35.1766, 22.2823)
  line L1657 (35.1766, 22.2823) -> (35.1586, 22.2733)
  line L1658 (35.1586, 22.2733) -> (35.1404, 22.2646)
  line L1659 (35.1404, 22.2646) -> (35.1219, 22.2562)
  line L1660 (35.1219, 22.2562) -> (35.1036, 22.2482)
  line L1661 (35.1036, 22.2482) -> (35.0848, 22.2405)
  line L1662 (35.0848, 22.2405) -> (35.066, 22.2331)
  line L1663 (35.066, 22.2331) -> (35.0472, 22.226)
  line L1664 (35.0472, 22.226) -> (35.0282, 22.2193)
  line L1665 (35.0282, 22.2193) -> (35.0091, 22.2129)
  line L1666 (35.0091, 22.2129) -> (34.9898, 22.2068)
  line L1667 (34.9898, 22.2068) -> (34.9705, 22.2011)
  line L1668 (34.9705, 22.2011) -> (34.9512, 22.1957)
  line L1669 (34.9512, 22.1957) -> (34.9316, 22.1907)
  line L1670 (34.9316, 22.1907) -> (34.912, 22.186)
  line L1671 (34.912, 22.186) -> (34.8922, 22.1816)
  line L1672 (34.8922, 22.1816) -> (34.8726, 22.1776)
  line L1673 (34.8726, 22.1776) -> (34.8528, 22.1739)
  line L1674 (34.8528, 22.1739) -> (34.8329, 22.1706)
  line L1675 (34.8329, 22.1706) -> (34.8128, 22.1676)
  line L1676 (34.8128, 22.1676) -> (34.793, 22.165)
  line L1677 (34.793, 22.165) -> (34.7729, 22.1627)
  line L1678 (34.7729, 22.1627) -> (34.7528, 22.1608)
  line L1679 (34.7528, 22.1608) -> (34.7326, 22.1592)
  line L1680 (34.7326, 22.1592) -> (34.7125, 22.158)
  line L1681 (34.7125, 22.158) -> (34.6924, 22.1571)
  line L1682 (34.6924, 22.1571) -> (34.6723, 22.1566)
  line L1683 (34.6723, 22.1566) -> (34.6522, 22.1564)
  line L1684 (34.6522, 22.1564) -> (34.6321, 22.1566)
  line L1685 (3.7802, 6.0904) -> (3.7656, 6.0905)
  line L1686 (3.7656, 6.0905) -> (3.7509, 6.0909)
  line L1687 (3.7509, 6.0909) -> (3.7363, 6.0915)
  line L1688 (3.7363, 6.0915) -> (3.7216, 6.0924)
  line L1689 (3.7216, 6.0924) -> (3.707, 6.0936)
  line L1690 (3.707, 6.0936) -> (3.6924, 6.095)
  line L1691 (3.6924, 6.095) -> (3.6779, 6.0966)
  line L1692 (3.6779, 6.0966) -> (3.6633, 6.0985)
  line L1693 (3.6633, 6.0985) -> (3.6488, 6.1007)
  line L1694 (3.6488, 6.1007) -> (3.6344, 6.1031)
  line L1695 (3.6344, 6.1031) -> (3.6199, 6.1058)
  line L1696 (3.6199, 6.1058) -> (3.6056, 6.1087)
  line L1697 (3.6056, 6.1087) -> (3.5913, 6.1119)
  line L1698 (3.5913, 6.1119) -> (3.577, 6.1153)
  line L1699 (3.577, 6.1153) -> (3.5628, 6.119)
  line L1700 (3.5628, 6.119) -> (3.5487, 6.1229)
  line L1701 (3.5487, 6.1229) -> (3.5346, 6.1271)
  line L1702 (3.5346, 6.1271) -> (3.5207, 6.1315)
  line L1703 (3.5207, 6.1315) -> (3.5067, 6.1361)
  line L1704 (3.5067, 6.1361) -> (3.4929, 6.141)
  line L1705 (3.4929, 6.141) -> (3.4792, 6.1462)
  line L1706 (3.4792, 6.1462) -> (3.4655, 6.1515)
  line L1707 (3.4655, 6.1515) -> (3.452, 6.1571)
  line L1708 (3.452, 6.1571) -> (3.4386, 6.163)
  line L1709 (3.4386, 6.163) -> (3.4252, 6.1691)
  line L1710 (3.4252, 6.1691) -> (3.412, 6.1754)
  line L1711 (3.412, 6.1754) -> (3.3989, 6.1819)
  line L1712 (3.3989, 6.1819) -> (3.3858, 6.1887)
  line L1713 (3.3858, 6.1887) -> (3.373, 6.1957)
  line L1714 (3.373, 6.1957) -> (3.3602, 6.2029)
  line L1715 (3.3602, 6.2029) -> (3.3476, 6.2104)
  line L1716 (3.3476, 6.2104) -> (3.3351, 6.218)
  line L1717 (3.3351, 6.218) -> (3.3227, 6.2259)
  line L1718 (3.3227, 6.2259) -> (3.3105, 6.234)
  line L1719 (3.3105, 6.234) -> (3.2984, 6.2423)
  line L1720 (3.2984, 6.2423) -> (3.2865, 6.2508)
  line L1721 (3.2865, 6.2508) -> (3.2747, 6.2595)
  line L1722 (3.2747, 6.2595) -> (3.2631, 6.2685)
  line L1723 (3.2631, 6.2685) -> (3.2516, 6.2776)
  line L1724 (3.2516, 6.2776) -> (3.2402, 6.2869)
  line L1725 (3.2402, 6.2869) -> (3.2291, 6.2964)
  line L1726 (3.2291, 6.2964) -> (3.2181, 6.3062)
  line L1727 (3.2181, 6.3062) -> (3.2073, 6.3161)
  line L1728 (3.2073, 6.3161) -> (3.1967, 6.3261)
  line L1729 (3.1967, 6.3261) -> (3.1862, 6.3364)
  line L1730 (3.1862, 6.3364) -> (3.176, 6.3469)
  line L1731 (3.176, 6.3469) -> (3.1658, 6.3575)
  line L1732 (3.1658, 6.3575) -> (3.156, 6.3683)
  line L1733 (3.156, 6.3683) -> (3.1462, 6.3793)
  line L1734 (3.1462, 6.3793) -> (3.1367, 6.3905)
  line L1735 (3.1367, 6.3905) -> (3.1274, 6.4018)
  line L1736 (3.1274, 6.4018) -> (3.1183, 6.4132)
  line L1737 (3.1183, 6.4132) -> (3.1093, 6.4249)
  line L1738 (3.1093, 6.4249) -> (3.1006, 6.4367)
  line L1739 (3.1006, 6.4367) -> (3.0921, 6.4486)
  line L1740 (3.0921, 6.4486) -> (3.0838, 6.4607)
  line L1741 (3.0838, 6.4607) -> (3.0757, 6.4729)
  line L1742 (3.0757, 6.4729) -> (3.0678, 6.4853)
  line L1743 (3.0678, 6.4853) -> (3.0602, 6.4978)
  line L1744 (3.0602, 6.4978) -> (3.0527, 6.5104)
  line L1745 (3.0527, 6.5104) -> (3.0455, 6.5232)
  line L1746 (3.0455, 6.5232) -> (3.0385, 6.5361)
  line L1747 (3.0385, 6.5361) -> (3.0317, 6.549)
  line L1748 (3.0317, 6.549) -> (3.0252, 6.5622)
  line L1749 (3.0252, 6.5622) -> (3.0189, 6.5754)
  line L1750 (3.0189, 6.5754) -> (3.0128, 6.5888)
  line L1751 (3.0128, 6.5888) -> (3.007, 6.6022)
  line L1752 (3.007, 6.6022) -> (3.0014, 6.6157)
  line L1753 (3.0014, 6.6157) -> (2.996, 6.6294)
  line L1754 (2.996, 6.6294) -> (2.9908, 6.6431)
  line L1755 (2.9908, 6.6431) -> (2.986, 6.6569)
  line L1756 (2.986, 6.6569) -> (2.9813, 6.6708)
  line L1757 (2.9813, 6.6708) -> (2.9769, 6.6848)
  line L1758 (2.9769, 6.6848) -> (2.9727, 6.6989)
  line L1759 (2.9727, 6.6989) -> (2.9688, 6.713)
  line L1760 (2.9688, 6.713) -> (2.9651, 6.7272)
  line L1761 (2.9651, 6.7272) -> (2.9617, 6.7415)
  line L1762 (2.9617, 6.7415) -> (2.9585, 6.7558)
  line L1763 (2.9585, 6.7558) -> (2.9556, 6.7701)
  line L1764 (2.9556, 6.7701) -> (2.9529, 6.7846)
  line L1765 (2.9529, 6.7846) -> (2.9505, 6.799)
  line L1766 (2.9505, 6.799) -> (2.9484, 6.8135)
  line L1767 (2.9484, 6.8135) -> (2.9465, 6.828)
  line L1768 (2.9465, 6.828) -> (2.9448, 6.8426)
  line L1769 (2.9448, 6.8426) -> (2.9434, 6.8572)
  line L1770 (2.9434, 6.8572) -> (2.9422, 6.8718)
  line L1771 (2.9422, 6.8718) -> (2.9413, 6.8865)
  line L1772 (2.9413, 6.8865) -> (2.9407, 6.9011)
  line L1773 (2.9407, 6.9011) -> (2.9403, 6.9158)
  line L1774 (2.9403, 6.9158) -> (2.9402, 6.9304)
  line L1775 (2.9402, 6.9304) -> (2.9402, 17.8511)
  line L1776 (2.9402, 17.8511) -> (2.9403, 17.8658)
  line L1777 (2.9403, 17.8658) -> (2.9407, 17.8804)
  line L1778 (2.9407, 17.8804) -> (2.9413, 17.8951)
  line L1779 (2.9413, 17.8951) -> (2.9422, 17.9097)
  line L1780 (2.9422, 17.9097) -> (2.9434, 17.9243)
  line L1781 (2.9434, 17.9243) -> (2.9448, 17.9389)
  line L1782 (2.9448, 17.9389) -> (2.9465, 17.9535)
  line L1783 (2.9465, 17.9535) -> (2.9484, 17.968)
  line L1784 (2.9484, 17.968) -> (2.9505, 17.9825)
  line L1785 (2.9505, 17.9825) -> (2.9529, 17.997)
  line L1786 (2.9529, 17.997) -> (2.9556, 18.0114)
  line L1787 (2.9556, 18.0114) -> (2.9585, 18.0258)
  line L1788 (2.9585, 18.0258) -> (2.9617, 18.0401)
  line L1789 (2.9617, 18.0401) -> (2.9651, 18.0543)
  line L1790 (2.9651, 18.0543) -> (2.9688, 18.0685)
  line L1791 (2.9688, 18.0685) -> (2.9727, 18.0827)
  line L1792 (2.9727, 18.0827) -> (2.9769, 18.0967)
  line L1793 (2.9769, 18.0967) -> (2.9813, 18.1107)
  line L1794 (2.9813, 18.1107) -> (2.986, 18.1246)
  line L1795 (2.986, 18.1246) -> (2.9908, 18.1384)
  line L1796 (2.9908, 18.1384) -> (2.996, 18.1522)
  line L1797 (2.996, 18.1522) -> (3.0014, 18.1658)
  line L1798 (3.0014, 18.1658) -> (3.007, 18.1793)
  line L1799 (3.007, 18.1793) -> (3.0128, 18.1928)
  line L1800 (3.0128, 18.1928) -> (3.0189, 18.2061)
  line L1801 (3.0189, 18.2061) -> (3.0252, 18.2194)
  line L1802 (3.0252, 18.2194) -> (3.0317, 18.2325)
  line L1803 (3.0317, 18.2325) -> (3.0385, 18.2455)
  line L1804 (3.0385, 18.2455) -> (3.0455, 18.2584)
  line L1805 (3.0455, 18.2584) -> (3.0527, 18.2711)
  line L1806 (3.0527, 18.2711) -> (3.0602, 18.2838)
  line L1807 (3.0602, 18.2838) -> (3.0678, 18.2963)
  line L1808 (3.0678, 18.2963) -> (3.0757, 18.3086)
  line L1809 (3.0757, 18.3086) -> (3.0838, 18.3209)
  line L1810 (3.0838, 18.3209) -> (3.0921, 18.3329)
  line L1811 (3.0921, 18.3329) -> (3.1006, 18.3449)
  line L1812 (3.1006, 18.3449) -> (3.1093, 18.3567)
  line L1813 (3.1093, 18.3567) -> (3.1183, 18.3683)
  line L1814 (3.1183, 18.3683) -> (3.1274, 18.3798)
  line L1815 (3.1274, 18.3798) -> (3.1367, 18.3911)
  line L1816 (3.1367, 18.3911) -> (3.1462, 18.4022)
  line L1817 (3.1462, 18.4022) -> (3.156, 18.4132)
  line L1818 (3.156, 18.4132) -> (3.1658, 18.424)
  line L1819 (3.1658, 18.424) -> (3.176, 18.4347)
  line L1820 (3.176, 18.4347) -> (3.1862, 18.4451)
  line L1821 (3.1862, 18.4451) -> (3.1967, 18.4554)
  line L1822 (3.1967, 18.4554) -> (3.2073, 18.4655)
  line L1823 (3.2073, 18.4655) -> (3.2181, 18.4754)
  line L1824 (3.2181, 18.4754) -> (3.2291, 18.4851)
  line L1825 (3.2291, 18.4851) -> (3.2402, 18.4946)
  line L1826 (3.2402, 18.4946) -> (3.2516, 18.504)
  line L1827 (3.2516, 18.504) -> (3.2631, 18.5131)
  line L1828 (3.2631, 18.5131) -> (3.2747, 18.522)
  line L1829 (3.2747, 18.522) -> (3.2865, 18.5307)
  line L1830 (3.2865, 18.5307) -> (3.2984, 18.5392)
  line L1831 (3.2984, 18.5392) -> (3.3105, 18.5475)
  line L1832 (3.3105, 18.5475) -> (3.3227, 18.5556)
  line L1833 (3.3227, 18.5556) -> (3.3351, 18.5635)
  line L1834 (3.3351, 18.5635) -> (3.3476, 18.5712)
  line L1835 (3.3476, 18.5712) -> (3.3602, 18.5786)
  line L1836 (3.3602, 18.5786) -> (3.373, 18.5858)
  line L1837 (3.373, 18.5858) -> (3.3858, 18.5928)
  line L1838 (3.3858, 18.5928) -> (3.3989, 18.5996)
  line L1839 (3.3989, 18.5996) -> (3.412, 18.6061)
  line L1840 (3.412, 18.6061) -> (3.4252, 18.6125)
  line L1841 (3.4252, 18.6125) -> (3.4386, 18.6185)
  line L1842 (3.4386, 18.6185) -> (3.452, 18.6244)
  line L1843 (3.452, 18.6244) -> (3.4655, 18.63)
  line L1844 (3.4655, 18.63) -> (3.4792, 18.6354)
  line L1845 (3.4792, 18.6354) -> (3.4929, 18.6405)
  line L1846 (3.4929, 18.6405) -> (3.5067, 18.6454)
  line L1847 (3.5067, 18.6454) -> (3.5207, 18.65)
  line L1848 (3.5207, 18.65) -> (3.5346, 18.6544)
  line L1849 (3.5346, 18.6544) -> (3.5487, 18.6586)
  line L1850 (3.5487, 18.6586) -> (3.5628, 18.6625)
  line L1851 (3.5628, 18.6625) -> (3.577, 18.6662)
  line L1852 (3.577, 18.6662) -> (3.5913, 18.6696)
  line L1853 (3.5913, 18.6696) -> (3.6056, 18.6728)
  line L1854 (3.6056, 18.6728) -> (3.6199, 18.6757)
  line L1855 (3.6199, 18.6757) -> (3.6344, 18.6784)
  line L1856 (3.6344, 18.6784) -> (3.6488, 18.6808)
  line L1857 (3.6488, 18.6808) -> (3.6633, 18.683)
  line L1858 (3.6633, 18.683) -> (3.6779, 18.6849)
  line L1859 (3.6779, 18.6849) -> (3.6924, 18.6865)
  line L1860 (3.6924, 18.6865) -> (3.707, 18.688)
  line L1861 (3.707, 18.688) -> (3.7216, 18.6891)
  line L1862 (3.7216, 18.6891) -> (3.7363, 18.69)
  line L1863 (3.7363, 18.69) -> (3.7509, 18.6906)
  line L1864 (3.7509, 18.6906) -> (3.7656, 18.691)
  line L1865 (3.7656, 18.691) -> (3.7802, 18.6911)
  line L1866 (3.7802, 18.6911) -> (31.0819, 18.6911)
  line L1867 (31.0819, 18.6911) -> (31.0965, 18.691)
  line L1868 (31.0965, 18.691) -> (31.1113, 18.6906)
  line L1869 (31.1113, 18.6906) -> (31.1258, 18.69)
  line L1870 (31.1258, 18.69) -> (31.1404, 18.6891)
  line L1871 (31.1404, 18.6891) -> (31.1552, 18.688)
  line L1872 (31.1552, 18.688) -> (31.1698, 18.6865)
  line L1873 (31.1698, 18.6865) -> (31.1843, 18.6849)
  line L1874 (31.1843, 18.6849) -> (31.1989, 18.683)
  line L1875 (31.1989, 18.683) -> (31.2134, 18.6808)
  line L1876 (31.2134, 18.6808) -> (31.2277, 18.6784)
  line L1877 (31.2277, 18.6784) -> (31.2423, 18.6757)
  line L1878 (31.2423, 18.6757) -> (31.2566, 18.6728)
  line L1879 (31.2566, 18.6728) -> (31.2708, 18.6696)
  line L1880 (31.2708, 18.6696) -> (31.2851, 18.6662)
  line L1881 (31.2851, 18.6662) -> (31.2994, 18.6625)
  line L1882 (31.2994, 18.6625) -> (31.3134, 18.6586)
  line L1883 (31.3134, 18.6586) -> (31.3275, 18.6544)
  line L1884 (31.3275, 18.6544) -> (31.3415, 18.65)
  line L1885 (31.3415, 18.65) -> (31.3555, 18.6454)
  line L1886 (31.3555, 18.6454) -> (31.3693, 18.6405)
  line L1887 (31.3693, 18.6405) -> (31.383, 18.6354)
  line L1888 (31.383, 18.6354) -> (31.3965, 18.63)
  line L1889 (31.3965, 18.63) -> (31.4103, 18.6244)
  line L1890 (31.4103, 18.6244) -> (31.4235, 18.6185)
  line L1891 (31.4235, 18.6185) -> (31.437, 18.6125)
  line L1892 (31.437, 18.6125) -> (31.4502, 18.6061)
  line L1893 (31.4502, 18.6061) -> (31.4632, 18.5996)